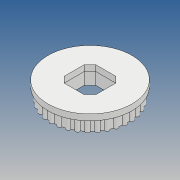
# Autodesk Inventor part: engrane correa dado-motor 2
Saved by Autodesk Inventor 2017 (Build 210142000, 142)
## iProperties
Part Number: engrane correa dado-motor 2
Material: Genérico
Document SubType Name: Modeling
Designer: FABLAB
Density: 1 g/cm^3
Appearance: Blanco
Description: Acrílico corte laser CNC
Author: FABLAB
Autodesk Inventor part; units mm, degrees
ref_plane "YZ Plane" through (0, 0, 0) normal (1, 0, 0) x (0, 1, 0)
ref_plane "XZ Plane" through (0, 0, 0) normal (0, 1, 0) x (-1, 0, 0)
ref_plane "XY Plane" through (0, 0, 0) normal (0, 0, 1) x (1, 0, 0)
sketch "Boceto1" plane through (0, 0, 0) normal (0, 0, 1) x (1, 0, 0)
  line L0 (8, -8) -> (-8, -8) projected
  line L1 (-8, -8) -> (-8, 8) projected
  line L2 (-8, 8) -> (8, 8) projected
  line L3 (8, 8) -> (8, -8) projected
  circle A0 centre (0, 0) radius 15 construction
  circle A1 centre (0, 0) radius 19.155
  circle A2 centre (0, 0) radius 16.155 construction
  circle A3 centre (0, 16.155) radius 1.25
  circle A4 centre (0, -16.155) radius 1.25
  circle A5 centre (0, 19.155) radius 1
  circle A6 centre (-3.5197, 18.8288) radius 1
  circle A7 centre (-6.9196, 17.8615) radius 1
  circle A8 centre (-10.0838, 16.2859) radius 1
  circle A9 centre (-12.9046, 14.1557) radius 1
  circle A10 centre (-15.286, 11.5435) radius 1
  circle A11 centre (-17.1469, 8.5381) radius 1
  circle A12 centre (-18.4238, 5.242) radius 1
  circle A13 centre (-19.0733, 1.7674) radius 1
  circle A14 centre (-19.0733, -1.7674) radius 1
  circle A15 centre (-18.4238, -5.242) radius 1
  circle A16 centre (-17.1469, -8.5381) radius 1
  circle A17 centre (-15.286, -11.5435) radius 1
  circle A18 centre (-12.9046, -14.1557) radius 1
  circle A19 centre (-10.0838, -16.2859) radius 1
  circle A20 centre (-6.9196, -17.8615) radius 1
  circle A21 centre (-3.5197, -18.8288) radius 1
  circle A22 centre (0, -19.155) radius 1
  circle A23 centre (3.5197, -18.8288) radius 1
  circle A24 centre (6.9196, -17.8615) radius 1
  circle A25 centre (10.0838, -16.2859) radius 1
  circle A26 centre (12.9046, -14.1557) radius 1
  circle A27 centre (15.286, -11.5435) radius 1
  circle A28 centre (17.1469, -8.5381) radius 1
  circle A29 centre (18.4238, -5.242) radius 1
  circle A30 centre (19.0733, -1.7674) radius 1
  circle A31 centre (19.0733, 1.7674) radius 1
  circle A32 centre (18.4238, 5.242) radius 1
  circle A33 centre (17.1469, 8.5381) radius 1
  circle A34 centre (15.286, 11.5435) radius 1
  circle A35 centre (0, 0) radius 21.655 construction
  circle A36 centre (12.9046, 14.1557) radius 1
  circle A37 centre (10.0838, 16.2859) radius 1
  circle A38 centre (6.9196, 17.8615) radius 1
  circle A39 centre (3.5197, 18.8288) radius 1
  dimension "d0" = 38.31
  dimension "d4" = 3
  dimension "d3" = 2.5
  dimension "d7" = 360
  dimension "d16" = 2
  dimension "d19" = 360
  dimension "d24" = 43.31
  dimension "d25" = 3.5348
  dimension "d27" = 2.5
  constraints: 37 centre point, 4 vertical alignment, 3 coincident, 78 other
  measures "d3" diameter of A3
  measures "d16" diameter of A5
  measures "d24" diameter of A35
  measures "d25" distance of A31.centre A32.centre
extrude "Extrusión1" add sketch "Boceto1" along normal blind 6 contours A1 A30 A29 A28 A27 A26 A25 A24 A23 A22 A21 A20 A19 A18 A17 A16 A15 A14 A13 A12 A11 A10 A9 A8 A7 A6 A5 A39 A38 A37 A36 A34 A33 A32 A31 | A31 A1 | A1 A31 | A30 A1 | A1 A30 | A32 A1 | A1 A32 | A29 A1 | A1 A29 | A33 A1 | A1 A33 | A28 A1 | A1 A28 | A34 A1 | A1 A34 | A27 A1 | A1 A27 | A36 A1 | A1 A36 | A26 A1 | A1 A26 | A37 A1 | A1 A37 | A25 A1 | A1 A25 | A38 A1 | A1 A38 | A24 A1 | A1 A24 | A39 A1 | A1 A39 | A23 A1 | A1 A23 | A5 A1 | A1 A5 | A22 A1 | A1 A22 | A6 A1 | A1 A6 | A21 A1 | A1 A21 | A7 A1 | A1 A7 | A20 A1 | A1 A20 | A8 A1 | A1 A8 | A19 A1 | A1 A19 | A9 A1 | A1 A9 | A18 A1 | A1 A18 | A10 A1 | A1 A10 | A17 A1 | A1 A17 | A11 A1 | A1 A11 | A16 A1 | A1 A16 | A12 A1 | A1 A12 | A15 A1 | A1 A15 | A13 A1 | A1 A13 | A14 A1 | A1 A14 | A3 | A4
chamfer "Chaflán1" distance 3 angle 45 4 edges at (-8, 8, 3) (8, 8, 3) (8, -8, 3) (-8, -8, 3)
sketch "Boceto3" plane through (0, 0, 6) normal (0, 0, 1) x (1, 0, 0)
  line L0 (-8, -5) -> (-8, 5) projected
  line L1 (-5, 8) -> (-8, 5) projected
  line L2 (-5, 8) -> (5, 8) projected
  line L3 (8, 5) -> (5, 8) projected
  line L4 (8, 5) -> (8, -5) projected
  line L5 (5, -8) -> (8, -5) projected
  line L6 (5, -8) -> (-5, -8) projected
  line L7 (-8, -5) -> (-5, -8) projected
  arc A0 (16.6779, 9.4213) -> (15.8676, 10.73) centre (0, 0) ccw construction
  arc A1 (15.8676, 10.73) -> (14.6628, 12.3255) centre (15.286, 11.5435) ccw construction
  arc A2 (14.6628, 12.3255) -> (13.6258, 13.463) centre (0, 0) ccw construction
  arc A3 (0.9997, 19.1289) -> (-0.9997, 19.1289) centre (0, 19.155) ccw construction
  arc A4 (-0.9997, 19.1289) -> (-2.5323, 18.9869) centre (0, 0) ccw construction
  arc A5 (-2.5323, 18.9869) -> (-4.4976, 18.6195) centre (-3.5197, 18.8288) ccw construction
  arc A6 (-4.4976, 18.6195) -> (-5.978, 18.1983) centre (0, 0) ccw construction
  arc A7 (-5.978, 18.1983) -> (-7.8423, 17.476) centre (-6.9196, 17.8615) ccw construction
  arc A8 (-7.8423, 17.476) -> (-9.2201, 16.79) centre (0, 0) ccw construction
  arc A9 (-9.2201, 16.79) -> (-10.92, 15.7375) centre (-10.0838, 16.2859) ccw construction
  arc A10 (-10.92, 15.7375) -> (-12.1483, 14.8099) centre (0, 0) ccw construction
  arc A11 (-12.1483, 14.8099) -> (-13.6258, 13.463) centre (-12.9046, 14.1557) ccw construction
  arc A12 (-13.6258, 13.463) -> (-14.6628, 12.3255) centre (0, 0) ccw construction
  arc A13 (-14.6628, 12.3255) -> (-15.8676, 10.73) centre (-15.286, 11.5435) ccw construction
  arc A14 (-15.8676, 10.73) -> (-16.6779, 9.4213) centre (0, 0) ccw construction
  arc A15 (-16.6779, 9.4213) -> (-17.5691, 7.6316) centre (-17.1469, 8.5381) ccw construction
  arc A16 (-17.5691, 7.6316) -> (-18.1251, 6.1964) centre (0, 0) ccw construction
  arc A17 (-18.1251, 6.1964) -> (-18.6722, 4.2734) centre (-18.4238, 5.242) ccw construction
  arc A18 (-18.6722, 4.2734) -> (-18.9551, 2.7604) centre (0, 0) ccw construction
  arc A19 (-18.9551, 2.7604) -> (-19.1395, 0.7696) centre (-19.0733, 1.7674) ccw construction
  arc A20 (-19.1395, 0.7696) -> (-19.1395, -0.7696) centre (0, 0) ccw construction
  arc A21 (-19.1395, -0.7696) -> (-18.9551, -2.7604) centre (-19.0733, -1.7674) ccw construction
  arc A22 (-18.9551, -2.7604) -> (-18.6722, -4.2734) centre (0, 0) ccw construction
  arc A23 (-18.6722, -4.2734) -> (-18.1251, -6.1964) centre (-18.4238, -5.242) ccw construction
  arc A24 (-18.1251, -6.1964) -> (-17.5691, -7.6316) centre (0, 0) ccw construction
  arc A25 (-17.5691, -7.6316) -> (-16.6779, -9.4213) centre (-17.1469, -8.5381) ccw construction
  arc A26 (-16.6779, -9.4213) -> (-15.8676, -10.73) centre (0, 0) ccw construction
  arc A27 (-15.8676, -10.73) -> (-14.6628, -12.3255) centre (-15.286, -11.5435) ccw construction
  arc A28 (-14.6628, -12.3255) -> (-13.6258, -13.463) centre (0, 0) ccw construction
  arc A29 (-13.6258, -13.463) -> (-12.1483, -14.8099) centre (-12.9046, -14.1557) ccw construction
  arc A30 (-12.1483, -14.8099) -> (-10.92, -15.7375) centre (0, 0) ccw construction
  arc A31 (-10.92, -15.7375) -> (-9.2201, -16.79) centre (-10.0838, -16.2859) ccw construction
  arc A32 (-9.2201, -16.79) -> (-7.8423, -17.476) centre (0, 0) ccw construction
  arc A33 (-7.8423, -17.476) -> (-5.978, -18.1983) centre (-6.9196, -17.8615) ccw construction
  arc A34 (-5.978, -18.1983) -> (-4.4976, -18.6195) centre (0, 0) ccw construction
  arc A35 (-4.4976, -18.6195) -> (-2.5323, -18.9869) centre (-3.5197, -18.8288) ccw construction
  arc A36 (-2.5323, -18.9869) -> (-0.9997, -19.1289) centre (0, 0) ccw construction
  arc A37 (-0.9997, -19.1289) -> (0.9997, -19.1289) centre (0, -19.155) ccw construction
  arc A38 (0.9997, -19.1289) -> (2.5323, -18.9869) centre (0, 0) ccw construction
  arc A39 (2.5323, -18.9869) -> (4.4976, -18.6195) centre (3.5197, -18.8288) ccw construction
  arc A40 (4.4976, -18.6195) -> (5.978, -18.1983) centre (0, 0) ccw construction
  arc A41 (5.978, -18.1983) -> (7.8423, -17.476) centre (6.9196, -17.8615) ccw construction
  arc A42 (7.8423, -17.476) -> (9.2201, -16.79) centre (0, 0) ccw construction
  arc A43 (9.2201, -16.79) -> (10.92, -15.7375) centre (10.0838, -16.2859) ccw construction
  arc A44 (10.92, -15.7375) -> (12.1483, -14.8099) centre (0, 0) ccw construction
  arc A45 (12.1483, -14.8099) -> (13.6258, -13.463) centre (12.9046, -14.1557) ccw construction
  arc A46 (13.6258, -13.463) -> (14.6628, -12.3255) centre (0, 0) ccw construction
  arc A47 (14.6628, -12.3255) -> (15.8676, -10.73) centre (15.286, -11.5435) ccw construction
  arc A48 (15.8676, -10.73) -> (16.6779, -9.4213) centre (0, 0) ccw construction
  arc A49 (16.6779, -9.4213) -> (17.5691, -7.6316) centre (17.1469, -8.5381) ccw construction
  arc A50 (17.5691, -7.6316) -> (18.1251, -6.1964) centre (0, 0) ccw construction
  arc A51 (18.1251, -6.1964) -> (18.6722, -4.2734) centre (18.4238, -5.242) ccw construction
  arc A52 (18.6722, -4.2734) -> (18.9551, -2.7604) centre (0, 0) ccw construction
  arc A53 (18.9551, -2.7604) -> (19.1395, -0.7696) centre (19.0733, -1.7674) ccw construction
  arc A54 (19.1395, -0.7696) -> (19.1395, 0.7696) centre (0, 0) ccw construction
  arc A55 (19.1395, 0.7696) -> (18.9551, 2.7604) centre (19.0733, 1.7674) ccw construction
  arc A56 (18.9551, 2.7604) -> (18.6722, 4.2734) centre (0, 0) ccw construction
  arc A57 (18.6722, 4.2734) -> (18.1251, 6.1964) centre (18.4238, 5.242) ccw construction
  arc A58 (18.1251, 6.1964) -> (17.5691, 7.6316) centre (0, 0) ccw construction
  arc A59 (17.5691, 7.6316) -> (16.6779, 9.4213) centre (17.1469, 8.5381) ccw construction
  circle A60 centre (0, 0) radius 21.155
  arc A61 (5.978, 18.1983) -> (4.4976, 18.6195) centre (0, 0) ccw projected
  arc A62 (4.4976, 18.6195) -> (2.5323, 18.9869) centre (3.5197, 18.8288) ccw projected
  arc A63 (2.5323, 18.9869) -> (0.9997, 19.1289) centre (0, 0) ccw projected
  arc A64 (13.6258, 13.463) -> (12.1483, 14.8099) centre (12.9046, 14.1557) ccw projected
  arc A65 (12.1483, 14.8099) -> (10.92, 15.7375) centre (0, 0) ccw projected
  arc A66 (10.92, 15.7375) -> (9.2201, 16.79) centre (10.0838, 16.2859) ccw projected
  arc A67 (9.2201, 16.79) -> (7.8423, 17.476) centre (0, 0) ccw projected
  arc A68 (7.8423, 17.476) -> (5.978, 18.1983) centre (6.9196, 17.8615) ccw projected
  dimension "d31" = 2
  constraints: 1 centre point, 1 coincident
  measures "d31" radial gap between concentric circles of A60 A58
extrude "Extrusión3" add sketch "Boceto3" along normal blind 3 separate body
